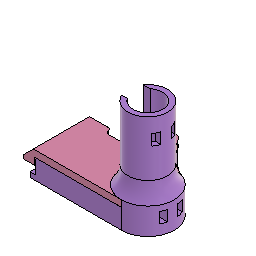
exit plate (Autodesk Fusion 360 design; units mm, degrees)
Autodesk Fusion 360 part; units mm, degrees
sketch "Sketch9" plane through (0, 0, 41.25) normal (0, 0, 1) x (-1, 0, 0)
  line L0 (20.7, -3.5) -> (19.2, -3.5)
  line L1 (19.2, -3.5) -> (19.2, -9)
  line L2 (19.2, -9) -> (27.7, -9)
  line L3 (27.7, -9) -> (27.7, -3.5)
  line L4 (27.7, -3.5) -> (20.7, -3.5)
  line L5 (27.7, -6.25) -> (19.2, -6.25) construction
  line L6 (24.2, -7.25) -> (19.2, -7.25)
  line L7 (19.2, -7.25) -> (19.2, -5.25)
  line L8 (19.2, -5.25) -> (24.2, -5.25)
  line L9 (24.2, -5.25) -> (24.2, -7.25)
  line L10 (24.2, 4.25) -> (19.2, 4.25)
  line L11 (19.2, 4.25) -> (19.2, 6.25)
  line L12 (19.2, 6.25) -> (24.2, 6.25)
  line L13 (24.2, 6.25) -> (24.2, 4.25)
  line L14 (19.2, -17.625) -> (19.2, 4)
  line L15 (19.2, -17.625) -> (19.2, -11.625) construction
  line L16 (19.2, -20.5) -> (19.2, -17.625) construction
  line L17 (19.2, -26.5) -> (19.2, -20.5) construction
  line L18 (19.2, -35.5) -> (19.2, -26.5) construction
  line L19 (19.2, -11.625) -> (19.2, 8) construction
  line L20 (27.7, -26.5) -> (27.7, -28) construction
  line L21 (27.7, -26.5) -> (27.7, -20.5) construction
  line L22 (27.7, -11.8) -> (27.7, -6) construction
  line L23 (27.7, -6) -> (27.7, 8) construction
  line L24 (19.2, 8) -> (27.7, 8) construction
  line L25 (27.7, -34) -> (27.7, -28) construction
  line L26 (27.7, -34) -> (27.7, -35.5) construction
  line L27 (27.7, -35.5) -> (19.2, -35.5) construction
  line L28 (27.7, -20.5) -> (27.7, -17.625)
  line L29 (27.7, -11.925) -> (27.7, -11.8)
  line L30 (27.7, -17.625) -> (27.7, -11.925)
  point P0 (19.2, 8)
  dimension "d1" = 2
  dimension "d2" = 5
  dimension "d3" = 1.75
  dimension "d4" = 1.75
  constraint midpoint L3 L5.start
  constraint midpoint L1 L5.end
  constraint horizontal L6
  constraint vertical L7
  constraint horizontal L8
  constraint vertical L9
  constraint midpoint L5.end L7
  constraint horizontal L10
  constraint vertical L11
  constraint horizontal L12
  constraint vertical L13
  constraint equal L9 L13
  constraint equal L6 L10
  constraint collinear L11 L14
  measures "d1" distance of L6.start L8.end
  measures "d2" distance of L6.end L9
  measures "d3" distance of L11.end P0
  measures "d4" vertical distance of L2.end L6.start
sketch "Sketch1" plane through (0, 0, 41.35) normal (0, 0, 1) x (-1, 0, 0)
  line L0 (20.7, 2.5) -> (27.7, 2.5)
  line L1 (27.7, 2.5) -> (27.7, 4)
  line L2 (27.7, 4) -> (21.7, 4)
  line L3 (19.2, -5) -> (27.7, -5)
  line L4 (27.7, -5) -> (27.7, -3.5)
  line L5 (16, 0) -> (0, 0) construction
  line L6 (27.7, 8) -> (27.7, -9)
  circle A0 centre (9.6, -14.775) radius 1.6
  circle A1 centre (9.6, -14.775) radius 1.65
  circle A2 centre (9.6, -14.775) radius 2.9
  circle A3 centre (0, 0) radius 6
  circle A4 centre (0, 0) radius 4.5
  line L7 (27.7, 2.5) -> (20.7, 2.5)
  line L8 (20.7, 2.5) -> (20.7, -3.5)
  line L9 (20.7, -3.5) -> (27.7, -3.5)
  line L10 (27.7, -3.5) -> (27.7, 2.5)
  line L11 (27.7, 8) -> (25.7, 8)
  line L12 (20.7, -3.5) -> (2.8284, -3.5)
  line L13 (20.7, 2.5) -> (3.7417, 2.5)
  line L14 (21.7, 8) -> (19.2, 8)
  circle A5 centre (0, 0) radius 8
  arc A6 (7.0735, -16.1986) -> (-2.9574, -7.4333) centre (-10.3509, -26.0165) ccw
  line L15 (0, 8) -> (27.7, 8)
  circle A7 centre (19, -0.5) radius 3
  line L16 (27.7, -3.5) -> (20.7, -3.5)
  line L17 (12.4791, -29.5958) -> (12.4791, -11.55)
  line L18 (12.4791, -11.55) -> (0.1, -11.55)
  line L19 (0.1, -11.55) -> (0.1, -11.8)
  line L20 (0.1, -11.8) -> (0.1438, -11.8)
  line L21 (0.1438, -11.8) -> (0.1438, -14.8)
  line L22 (0.1438, -14.8) -> (0.1, -14.8)
  line L23 (0.1, -14.8) -> (0.1, -18.05)
  line L24 (0.1, -18.05) -> (2.6, -18.05)
  line L25 (2.6, -18.05) -> (2.6, -19.3)
  line L26 (2.6, -19.3) -> (0.1, -19.3)
  line L27 (0.1, -19.3) -> (0.1, -24.5)
  arc A8 (0.1, -29.5) -> (0.1, -24.5) centre (0.1, -27) ccw
  line L28 (0.1, -29.5) -> (0.1, -29.5958)
  line L29 (0.1, -29.5958) -> (12.4791, -29.5958)
  circle A9 centre (9.6, -14.775) radius 1.6
  line L30 (12.5, -14.775) -> (12.5, -9.175)
  line L31 (14.5, -7.175) -> (19.1, -7.175)
  arc A10 (14.5, -7.175) -> (12.5, -9.175) centre (14.5, -9.175) ccw
  line L32 (27.7, -9) -> (21.1, -9)
  line L33 (20.1, -8) -> (20.1, -8.175)
  arc A11 (20.1, -8.175) -> (19.1, -7.175) centre (19.1, -8.175) ccw
  arc A12 (20.1, -8) -> (21.1, -9) centre (21.1, -8) ccw
  point P0 (12.5, -7.175)
  point P1 (20.1, -9)
  dimension "d450" = 5.8
  dimension "d451" = 4
  dimension "d452" = 4
  dimension "d453" = 12
  dimension "d454" = 9
  dimension "d562" = 16
  dimension "d580" = 3.3
  dimension "d581" = 7.6
  dimension "d582" = 2
  dimension "d583" = 7.6
  dimension "d584" = 1
  dimension "d585" = 1
  dimension "d586" = 20
  dimension "d657" = 19
  constraint coincident L5.end A3.centre
  constraint collinear L1 L6
  constraint concentric A0 A1
  constraint concentric A0 A2
  constraint horizontal L7
  constraint vertical L8
  constraint horizontal L9
  constraint vertical L10
  constraint coincident L8.end L9.start
  constraint coincident L0.end L1.start
  constraint perpendicular L6 L11
  constraint coincident L0.start L7.end
  constraint coincident A4 L12.end
  constraint coincident A4 L13.end
  constraint concentric A3 A5
  constraint tangent A2 A6
  constraint coincident A2 A6.start
  constraint coincident A5 A6.end
  constraint tangent A5 A6
  constraint coincident A5 L15.start
  constraint tangent A5 L15
  constraint coincident A2 L30.start
  constraint tangent A2 L30
  constraint perpendicular L6 L31
  constraint coincident P0 L30
  constraint coincident P0 L31
  constraint tangent L30 A10
  constraint tangent L31 A10
  constraint vertical L30
  constraint perpendicular L6 L32
  constraint perpendicular L31 L33
  constraint tangent L33 A11
  constraint tangent L31 A11
  constraint coincident P1 L33
  constraint coincident P1 L32
  constraint tangent L33 A12
  constraint tangent L32 A12
  constraint horizontal L5
  constraint horizontal L13
  constraint horizontal L12
  constraint tangent L12 A7
  constraint tangent L13 A7
  measures "d450" diameter of A2
  measures "d451" distance of L1.end L6.start
  measures "d452" distance of L3.end L6.end
  measures "d453" diameter of A3
  measures "d454" diameter of A4
  measures "d562" diameter of A5
  measures "d580" diameter of A1
  measures "d581" vertical distance of L30.start P0
  measures "d582" radius of A10
  measures "d583" distance of L6.end P1
  measures "d584" radius of A11
  measures "d585" radius of A12
  measures "d586" radius of A6
  measures "d657" horizontal distance of L5.end A7.centre
extrude "Extrude1" add sketch "Sketch1" along normal blind 6 contours L0 L1 L6 L7 L11 L13 L14 A5 L15 | L4 L6 A2 L9 L12 A5 A6 L16 L17 L18 L30 L31 A10 L32 L33 A11 A12 | A3 L12 L13 A5 | A3 A4 L12 L13 | A2 A6 L17 L18 | A2 L17 | A2 L17 picked at (5.7689, -4.4997) picked at (-4.3684, -3.3233) makes body 1
extrude "Extrude2" add sketch "Sketch1" along normal blind 30 contours A3 A4 L12 L13 picked at (-4.3684, -3.3233) bodies 1
extrude "Extrude7" add sketch "Sketch1" along normal blind 2 from surface at 6 contours A3 L12 L13 A5 picked at (5.7689, -4.4997) bodies 1
fillet "Fillet1" radius 8 1 edges at (5.9721, -0.5783, 49.35) on bodies 1
sketch "Sketch5" plane through (0, 0, 47.35) normal (0, 0, 1) x (-1, 0, 0)
  circle A0 centre (9.6, -14.775) radius 1.65
  line L0 (27.7, 8) -> (26.2, 8)
  line L1 (26.2, 8) -> (26.2, -9)
  line L2 (26.2, -9) -> (27.7, -9)
  line L3 (27.7, -9) -> (27.7, 8)
  line L4 (27.7, 8) -> (0, 8)
  arc A1 (-2.9574, -7.4333) -> (7.1937, -3.5) centre (0, 0) ccw
  arc A2 (7.0735, -16.1986) -> (-2.9574, -7.4333) centre (-10.3509, -26.0165) ccw
  arc A3 (7.0735, -16.1986) -> (12.5, -14.775) centre (9.6, -14.775) ccw
  line L5 (27.7, -9) -> (27.7, -3.5)
  line L6 (27.7, -3.5) -> (7.1937, -3.5)
  line L7 (12.5, -14.775) -> (12.5, -9.175)
  arc A4 (14.5, -7.175) -> (12.5, -9.175) centre (14.5, -9.175) ccw
  line L8 (14.5, -7.175) -> (19.1, -7.175)
  arc A5 (20.1, -8.175) -> (19.1, -7.175) centre (19.1, -8.175) ccw
  line L9 (20.1, -8.175) -> (20.1, -8)
  arc A6 (20.1, -8) -> (21.1, -9) centre (21.1, -8) ccw
  line L10 (21.1, -9) -> (27.7, -9)
  line L11 (27.7, 8) -> (27.7, -9)
  line L12 (19, -0.5) -> (19, 2.5)
  line L13 (19, 2.5) -> (19, -1.2273)
  line L14 (19, 0.387) -> (19, -3.5)
  circle A7 centre (19, -0.5) radius 3
  point P0 (19, -0.5)
  dimension "d528" = 1.5
  constraint horizontal L0
  constraint vertical L1
  constraint horizontal L2
  constraint vertical L3
  constraint collinear L0 L4
  constraint collinear L3 L11
  constraint vertical L12
  constraint coincident L12 L13.end
  constraint coincident L12 L14.start
  constraint vertical L14
  constraint coincident P0 L12.start
  constraint coincident L12.end A7
  constraint coincident L14.end A7
  measures "d528" distance of L0.start L0.end
extrude "Extrude6" add sketch "Sketch1" along normal blind 0.5 contours L12 L13 A5 A7 | A3 L12 L13 A5 | A3 A4 L12 L13 | A4 picked at (6.7742, -2.7851) picked at (5.172, 1.834) bodies 1
extrude "Extrude5" cut sketch "Sketch5" against normal blind 4.5 contours L0 L1 L3 L4 L6 L11 | L1 L2 L3 L5 L6 L10 L11 bodies 1
chamfer "Chamfer1" distance 0.5 angle 45 2 edges at (-26.2, 6.25, 47.35) (-26.2, -5.25, 47.35) on bodies 1
sketch "Sketch1 (2)" plane through (0, 0, 47.35) normal (0, 0, 1) x (-1, 0, 0) in component "exit cover"
  circle A0 centre (9.6, -14.775) radius 1.65
  circle A1 centre (0, 0) radius 4.5
  line L0 (25.2, -9) -> (26.3, -9)
  line L1 (25.2, 8) -> (26.3, 8)
  arc A2 (-2.9574, -7.4333) -> (7.1937, -3.5) centre (0, 0) ccw
  arc A3 (7.0735, -16.1986) -> (-2.9574, -7.4333) centre (-10.3509, -26.0165) ccw
  arc A4 (7.0735, -16.1986) -> (12.5, -14.775) centre (9.6, -14.775) ccw
  line L2 (25.7, 8) -> (0, 8)
  arc A5 (7.5993, 2.5) -> (0, 8) centre (0, 0) ccw
  circle A6 centre (0, 0) radius 8
  line L3 (3.7417, 2.5) -> (7.5993, 2.5)
  line L4 (2.8284, -3.5) -> (7.1937, -3.5)
  circle A7 centre (0, 0) radius 4.5
  arc A8 (7.5993, 2.5) -> (7.1937, -3.5) centre (0, 0) ccw
  arc A9 (5.4544, 2.5) -> (4.8734, -3.5) centre (0, 0) ccw
  line L5 (12.5, -14.775) -> (12.5, -9.175)
  arc A10 (14.5, -7.175) -> (12.5, -9.175) centre (14.5, -9.175) ccw
  line L6 (14.5, -7.175) -> (19.1, -7.175)
  arc A11 (20.1, -8.175) -> (19.1, -7.175) centre (19.1, -8.175) ccw
  line L7 (20.1, -8.175) -> (20.1, -8)
  arc A12 (20.1, -8) -> (21.1, -9) centre (21.1, -8) ccw
  line L8 (21.1, -9) -> (25.7, -9)
  line L9 (25.7, 8) -> (29.7, 8)
  line L10 (29.7, -9) -> (25.7, -9)
  line L11 (25.7, -9) -> (25.7, 8)
  line L12 (25.7, -9) -> (25.7, -3.5)
  line L13 (25.7, 2.5) -> (25.7, 8)
  line L14 (27.7, -9) -> (26.3, -9)
  line L15 (27.7, 8) -> (26.3, 8)
  line L16 (27.7, -17.625) -> (27.7, -9)
  line L17 (27.7, 8) -> (29.7, 8)
  line L18 (27.7, -20.5) -> (27.7, -17.625)
  line L19 (29.7, -20.5) -> (29.7, -17.625)
  line L20 (27.7, -20.5) -> (27.7, -26.5)
  line L21 (29.7, -26.5) -> (29.7, -20.5)
  line L22 (27.7, -35.5) -> (27.7, -26.5)
  line L23 (29.7, -35.5) -> (29.7, -26.5)
  line L24 (27.7, -35.5) -> (29.7, -35.5)
  line L25 (29.7, -9) -> (29.7, 8)
  line L26 (26.3, 8) -> (26.3, -9)
  dimension "d569" = 9
  dimension "d570" = 12
  constraint concentric A1 A6
  constraint concentric A2 A9
  constraint coincident A1 L3.start
  constraint coincident A5.start L3.end
  constraint coincident A1 L4.start
  constraint coincident A2.end L4.end
  constraint horizontal L4
  constraint horizontal L3
  constraint concentric A5 A7
  constraint coincident L3.start A7
  constraint concentric A7 A8
  constraint coincident L4 A9.end
  constraint coincident L3 A9.start
  constraint horizontal L9
  constraint horizontal L10
  constraint vertical L11
  constraint coincident L2.start L9.start
  constraint collinear L8 L10
  constraint perpendicular L17 L25
  constraint collinear L21 L25
  measures "d569" diameter of A1
  measures "d570" diameter of A9
extrude "Extrude1'" add sketch "Sketch1 (2)" along normal blind 2 separate body contours A1 A6 L3 L4 A7 | L0 L1 A2 A3 A4 L2 A5 A6 A8 L5 A10 L6 A11 L7 A12 L8 L11 L12 L13 | L0 L1 L9 L10 L11 L12 L13 L26 | L9 L10 L14 L15 L17 L25 L26 makes body 2 in component "exit cover"
sketch "Sketch2" plane through (0, 0, 47.35) normal (0, 0, -1) x (1, 0, 0) in component "exit cover"
  line L0 (-29.7, 8) -> (-26.4, 8)
  line L1 (-26.4, 8) -> (-26.4, -9)
  line L2 (-26.4, -9) -> (-29.7, -9)
  line L3 (-29.7, -9) -> (-29.7, 8)
  line L4 (-7.1937, -3.5) -> (-2.8284, -3.5)
  arc A0 (-3.7417, 2.5) -> (-2.8284, -3.5) centre (0, 0) ccw
  line L5 (-3.7417, 2.5) -> (-7.5993, 2.5)
  circle A1 centre (-9.6, -14.775) radius 1.65
  line L6 (-20.1, -8) -> (-20.1, -8.175)
  arc A2 (-19.1, -7.175) -> (-20.1, -8.175) centre (-19.1, -8.175) ccw
  line L7 (-19.1, -7.175) -> (-14.5, -7.175)
  arc A3 (-12.5, -9.175) -> (-14.5, -7.175) centre (-14.5, -9.175) ccw
  line L8 (-12.5, -9.175) -> (-12.5, -14.775)
  arc A4 (-12.5, -14.775) -> (-7.0735, -16.1986) centre (-9.6, -14.775) ccw
  arc A5 (2.9574, -7.4333) -> (-7.0735, -16.1986) centre (10.3509, -26.0165) ccw
  arc A6 (-7.1937, -3.5) -> (2.9574, -7.4333) centre (0, 0) ccw
  arc A7 (0, 8) -> (-7.5993, 2.5) centre (0, 0) ccw
  arc A8 (-21.1, -9) -> (-20.1, -8) centre (-21.1, -8) ccw
  line L9 (0, 8) -> (-29.7, 8)
  line L10 (-29.7, 8) -> (-29.7, -9)
  line L11 (-29.7, -9) -> (-21.1, -9)
  line L12 (-7.1937, -3.5) -> (-2.8284, -3.5)
  arc A9 (-3.7417, 2.5) -> (-2.8284, -3.5) centre (0, 0) ccw
  line L13 (-3.7417, 2.5) -> (-7.5993, 2.5)
  circle A10 centre (-9.6, -14.775) radius 1.65
  line L14 (-29.7, -9) -> (-21.1, -9)
  arc A11 (-21.1, -9) -> (-20.1, -8) centre (-21.1, -8) ccw
  line L15 (-20.1, -8) -> (-20.1, -8.175)
  arc A12 (-19.1, -7.175) -> (-20.1, -8.175) centre (-19.1, -8.175) ccw
  line L16 (-19.1, -7.175) -> (-14.5, -7.175)
  arc A13 (-12.5, -9.175) -> (-14.5, -7.175) centre (-14.5, -9.175) ccw
  line L17 (-12.5, -9.175) -> (-12.5, -14.775)
  arc A14 (-12.5, -14.775) -> (-7.0735, -16.1986) centre (-9.6, -14.775) ccw
  arc A15 (2.9574, -7.4333) -> (-7.0735, -16.1986) centre (10.3509, -26.0165) ccw
  arc A16 (-7.1937, -3.5) -> (2.9574, -7.4333) centre (0, 0) ccw
  arc A17 (0, 8) -> (-7.5993, 2.5) centre (0, 0) ccw
  line L18 (0, 8) -> (-29.7, 8)
  line L19 (-29.7, 8) -> (-29.7, -9)
  dimension "d558" = 3.3
  constraint horizontal L0
  constraint vertical L1
  constraint horizontal L2
  constraint vertical L3
  constraint collinear L3 L10
  measures "d558" distance of L1.end L2.end
extrude "Extrude2'" add sketch "Sketch2" along normal blind 2.1 contours L0 L1 L2 L3 L9 L10 L11 L14 L18 L19 bodies 2 in component "exit cover"
chamfer "Chamfer1'" distance 3 angle 45 1 edges at (-29.7, 0.5, 49.35) on bodies 2 in component "exit cover"
sketch "Sketch8" plane through (0, 0, 41.35) normal (0, 0, -1) x (1, 0, 0)
  line L0 (-20.7, -3.5) -> (-27.7, -3.5)
  line L1 (-27.7, -3.5) -> (-27.7, -9)
  line L2 (-27.7, -9) -> (-21.1, -9)
  arc A0 (-21.1, -9) -> (-20.1, -8) centre (-21.1, -8) ccw
  line L3 (-20.1, -8) -> (-20.1, -8.175)
  arc A1 (-19.1, -7.175) -> (-20.1, -8.175) centre (-19.1, -8.175) ccw
  line L4 (-19.1, -7.175) -> (-14.5, -7.175)
  arc A2 (-12.5, -9.175) -> (-14.5, -7.175) centre (-14.5, -9.175) ccw
  line L5 (-12.5, -9.175) -> (-12.5, -14.775)
  arc A3 (-12.5, -14.775) -> (-7.0735, -16.1986) centre (-9.6, -14.775) ccw
  arc A4 (2.9574, -7.4333) -> (-7.0735, -16.1986) centre (10.3509, -26.0165) ccw
  arc A5 (2.9574, -7.4333) -> (0, 8) centre (0, 0) ccw
  line L6 (0, 8) -> (-27.7, 8)
  line L7 (-27.7, 8) -> (-27.7, 2.5)
  line L8 (-27.7, 2.5) -> (-20.7, 2.5)
  arc A6 (-20.7, -3.5) -> (-20.7, 2.5) centre (-20.7, -0.5) ccw
  circle A7 centre (-9.6, -14.775) radius 1.65
  line L9 (-19, -3.5) -> (-27.7, -3.5)
  line L10 (-27.7, -3.5) -> (-27.7, -9)
  line L11 (-27.7, -9) -> (-21.1, -9)
  arc A8 (-21.1, -9) -> (-20.1, -8) centre (-21.1, -8) ccw
  line L12 (-20.1, -8) -> (-20.1, -8.175)
  arc A9 (-19.1, -7.175) -> (-20.1, -8.175) centre (-19.1, -8.175) ccw
  line L13 (-19.1, -7.175) -> (-14.5, -7.175)
  arc A10 (-12.5, -9.175) -> (-14.5, -7.175) centre (-14.5, -9.175) ccw
  line L14 (-12.5, -9.175) -> (-12.5, -14.775)
  arc A11 (-12.5, -14.775) -> (-7.0735, -16.1986) centre (-9.6, -14.775) ccw
  arc A12 (2.9574, -7.4333) -> (-7.0735, -16.1986) centre (10.3509, -26.0165) ccw
  arc A13 (2.9574, -7.4333) -> (0, 8) centre (0, 0) ccw
  line L15 (0, 8) -> (-27.7, 8)
  line L16 (-27.7, 8) -> (-27.7, 2.5)
  line L17 (-27.7, 2.5) -> (-19, 2.5)
  arc A14 (-19, -3.5) -> (-19, 2.5) centre (-19, -0.5) ccw
  circle A15 centre (-9.6, -14.775) radius 1.65
extrude "Extrude8" cut sketch "Sketch9" along normal blind 2.5 contours L10 L11 L12 L13 bodies 1
sketch "sketch 3120" plane through (0, 0, 0) normal (1, 0, 0) x (0, 1, 0)
  line L0 (-1.7834, 44.35) -> (-3.5834, 44.35)
  line L1 (-1.7834, 47.65) -> (-1.7834, 44.35)
  line L2 (-3.5834, 47.65) -> (-1.7834, 47.65)
  line L3 (-3.5834, 44.35) -> (-3.5834, 47.65)
  line L4 (-1.7834, 63.65) -> (-3.5834, 63.65)
  line L5 (-1.7834, 66.95) -> (-1.7834, 63.65)
  line L6 (-3.5834, 66.95) -> (-1.7834, 66.95)
  line L7 (-3.5834, 63.65) -> (-3.5834, 66.95)
  line L8 (3.0166, 63.65) -> (1.2166, 63.65)
  line L9 (3.0166, 66.95) -> (3.0166, 63.65)
  line L10 (1.2166, 66.95) -> (3.0166, 66.95)
  line L11 (1.2166, 63.65) -> (1.2166, 66.95)
  line L12 (3.0166, 44.35) -> (1.2166, 44.35)
  line L13 (3.0166, 47.65) -> (3.0166, 44.35)
  line L14 (1.2166, 47.65) -> (3.0166, 47.65)
  line L15 (1.2166, 44.35) -> (1.2166, 47.65)
extrude "Extrude9" cut sketch "sketch 3120" along normal through all bodies 1
component "exit cover" placed x (1, 0, 0) y (0, 1, 0) z (0, 0, 1) at (0, 0, 0)
named bodies: "exit plate", "exit cover"
